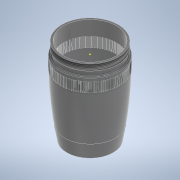
# Autodesk Inventor part: Top
Saved by Autodesk Inventor 2021 (Build 250183000, 183)
## iProperties
Created: 2020-04-07
Part Number: Top
Material: Generic
Document SubType Name: Modeling
Designer: Elijah
Density: 1 g/cm^3
Appearance: Silicon Nitride - Polished
Author: Elijah
Autodesk Inventor part; units mm, degrees
ref_plane "XZ Plane" through (0, 0, 0) normal (0, 1, 0) x (-1, 0, 0)
ref_plane "XY Plane" through (0, 0, 0) normal (0, 0, 1) x (1, 0, 0)
sketch "Sketch1" plane through (0, 0, 0) normal (0, 0, 1) x (1, 0, 0)
  line L0 (0, 0) -> (21.59, 0) construction
  line L1 (0, 0) -> (-9.5, 0)
  line L2 (0, 0) -> (0, 30)
  line L3 (0, 30) -> (-12, 30)
  line L4 (0, 30) -> (30.48, 30) construction
  arc A0 (-12, 30) -> (-9.5, 0) centre (145.7731, 28.0436) ccw
  dimension "d0" = 21.59
  dimension "d1" = 9.5
  dimension "d3" = 12
  dimension "d4" = 30.48
  dimension "d21" = 30
  constraints: 10 end point, 3 horizontal, 2 point on circle, 1 centre point, 1 perpendicular, 1 vertical
  measures "d0" distance of L0.start L0.end
  measures "d1" distance of L0.start L1.end
  measures "d3" distance of L2.end L3.end
  measures "d4" distance of L2.end L4.end
  measures "d21" vertical distance of L1.end L3.end
revolve "Revolution1" add sketch "Sketch1" angle 360 about axis through (0, 0, 0) along (0, 1, 0)
sketch "Sketch2" plane through (0, 30, 0) normal (0, 1, 0) x (1, 0, 0)
  point P0 (0, 0)
ref_plane "Work Plane1" through (41.275, 0, 0) normal (1, 0, 0) x (0, 1, 0)
sketch "Sketch6" plane through (41.275, 0, 0) normal (1, 0, 0) x (0, 1, 0)
  line L0 (28.8082, 0) -> (24.8082, 0)
  line L1 (24.8082, 0) -> (24.8082, -0.254)
  line L2 (24.8082, -0.254) -> (28.8082, -0.254)
  line L3 (28.8082, -0.254) -> (28.8082, 0)
  point P0 (0, 0)
  dimension "d22" = 4
  dimension "d23" = 0.254
  constraints: 8 end point, 2 parallel, 1 horizontal, 1 perpendicular
  measures "d22" distance of L2.end L1.end
  measures "d23" distance of L1.end L0.end
emboss "Emboss2" sketch "Sketch6" operation cut depth 1.27 direction (-1, 0, 0)
pattern_circular "Circular Pattern2" count 135 over 360 about axis through (0, 28.0436, 0) along (0, 1, 0) of "Emboss2"
sketch "Sketch7" plane through (0, 30, 0) normal (0, 1, 0) x (1, 0, 0)
  circle A0 centre (0, 0) radius 11.5
  dimension "d29" = 23
  constraints: 1 centre point, 1 coincident
  measures "d29" diameter of A0
extrude "Extrusion3" add sketch "Sketch7" along normal blind 0.2
sketch "Sketch8" plane through (0, 30.2, 0) normal (0, 1, 0) x (1, 0, 0)
  circle A0 centre (0, 0) radius 11
  dimension "d32" = 22
  constraints: 1 centre point, 1 coincident
  measures "d32" diameter of A0
extrude "Extrusion4" add sketch "Sketch8" along normal blind 2
sketch "Sketch9" plane through (0, 32.2, 0) normal (0, 1, 0) x (1, 0, 0)
  circle A0 centre (0, 0) radius 11.5
  dimension "d35" = 23
  constraints: 1 centre point, 1 coincident
  measures "d35" diameter of A0
extrude "Extrusion5" add sketch "Sketch9" along normal blind 2.6
thread "Thread2" size "M2.2x0.45" class "6g" standard "ISO Metric profile" full length
thread "Thread3" size "15/16-9 UNC" class "2A" standard "ANSI Unified Screw Threads" full length
sketch "Sketch10" plane through (0, 34.8, 0) normal (0, 1, 0) x (1, 0, 0)
  circle A0 centre (0, 0) radius 10.7087
  constraints: 1 centre point, 1 coincident
extrude "Extrusion6" cut sketch "Sketch10" against normal blind 25.4
sketch "Sketch11" plane through (0, 0, 0) normal (0, -1, 0) x (1, 0, 0)
  circle A0 centre (0, 0) radius 8.7741
  constraints: 1 centre point, 1 coincident
extrude "Extrusion7" cut sketch "Sketch11" against normal blind 12.7
sketch "Sketch12" plane through (0, 9.4, 0) normal (0, 1, 0) x (1, 0, 0)
  circle A0 centre (0, 0) radius 10.3883
  constraints: 1 centre point, 1 coincident
extrude "Extrusion8" cut sketch "Sketch12" against normal mid plane 7.62
body "Solid1"
